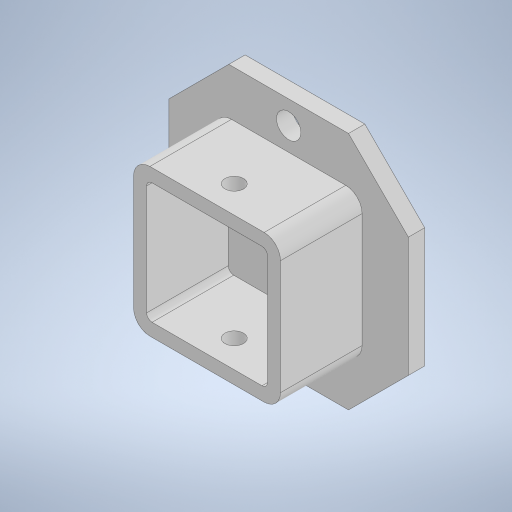
# Autodesk Inventor part: rod_fixture_vp16
Saved by Autodesk Inventor 2024 (Build 280153000, 153)
## iProperties
Created: 2024-10-07
Part Number: rod_fixture_vp16
Material: 一般
Document SubType Name: Modeling
Designer: 1412z
Density: 1 g/cm^3
Appearance: 既定
Author: 1412z
Autodesk Inventor part; units mm, degrees
ref_plane "YZ Plane" through (0, 0, 0) normal (1, 0, 0) x (0, 1, 0)
ref_plane "XZ Plane" through (0, 0, 0) normal (0, 1, 0) x (-1, 0, 0)
ref_plane "XY Plane" through (0, 0, 0) normal (0, 0, 1) x (1, 0, 0)
sketch "スケッチ1" plane through (0, 0, 0) normal (1, 0, 0) x (0, 1, 0)
  point P0 (0, 0)
sketch "スケッチ2" plane through (0, 0, 0) normal (0, 0, 1) x (1, 0, 0)
  line L0 (-11.1, 11.1) -> (11.1, 11.1)
  line L1 (11.1, 11.1) -> (11.1, -11.1)
  line L2 (11.1, -11.1) -> (-11.1, -11.1)
  line L3 (-11.1, -11.1) -> (-11.1, 11.1)
  line L4 (-11.1, 11.1) -> (11.1, -11.1) construction
  line L5 (11.1, 11.1) -> (-11.1, -11.1) construction
  line L6 (-13.5, -13.5) -> (13.5, -13.5)
  line L7 (13.5, -13.5) -> (13.5, 13.5)
  line L8 (13.5, 13.5) -> (-13.5, 13.5)
  line L9 (-13.5, 13.5) -> (-13.5, -13.5)
  line L10 (-13.5, -13.5) -> (13.5, 13.5) construction
  line L11 (13.5, -13.5) -> (-13.5, 13.5) construction
  point P0 (0, 0)
  dimension "d0" = 22.2
  dimension "d1" = 22.2
  dimension "d2" = 27
  dimension "d3" = 27
  constraints: 24 end point, 4 midpoint, 4 parallel, 2 horizontal, 2 perpendicular
  measures "d0" distance of L1.end L2.end
  measures "d1" distance of L0.end L1.end
  measures "d2" distance of L8.end L7.end
  measures "d3" distance of L7.end L6.end
extrude "押し出し1" add sketch "スケッチ2" along normal blind 15
sketch "スケッチ3" plane through (-13.5, 13.5, 0) normal (0, 1, 0) x (1, 0, 0)
  circle A0 centre (13.5, -10) radius 1.7
  point P0 (13.5, 0)
  dimension "d6" = 3.4
  constraints: 1 centre point
  measures "d6" diameter of A0
extrude "押し出し2" cut sketch "スケッチ3" against normal blind 30
sketch "スケッチ4" plane through (0, 0, 0) normal (0, 0, -1) x (-1, 0, 0)
  line L0 (22, 22) -> (-22, 22)
  line L1 (-22, 22) -> (-22, -22)
  line L2 (-22, -22) -> (22, -22)
  line L3 (22, -22) -> (22, 22)
  line L4 (22, 22) -> (-22, -22) construction
  line L5 (-22, 22) -> (22, -22) construction
  point P0 (0, 0)
  dimension "d9" = 44
  dimension "d10" = 44
  constraints: 12 end point, 2 midpoint, 2 parallel, 1 horizontal, 1 perpendicular
  measures "d9" distance of L2.end L1.end
  measures "d10" distance of L1.end L0.end
extrude "押し出し3" add sketch "スケッチ4" along normal blind 3
sketch "スケッチ5" plane through (0, 0, 0) normal (0, 0, 1) x (1, 0, 0)
  circle A0 centre (0, 17.75) radius 2.25
  circle A1 centre (0, -17.75) radius 2.25
  point P0 (0, 0)
  dimension "d13" = 4.5
  dimension "d14" = 4.5
  constraints: 2 centre point
  measures "d13" diameter of A0
  measures "d14" diameter of A1
extrude "押し出し4" cut sketch "スケッチ5" against normal blind 3
sketch "スケッチ6" plane through (0, 0, 0) normal (0, 0, 1) x (1, 0, 0)
  line L0 (-22, 22) -> (22, 22) projected
  line L1 (22, 22) -> (11, 22)
  line L2 (22, 22) -> (22, 11)
  line L3 (22, 11) -> (11, 22)
  line L4 (22, -22) -> (-22, -22) projected
  line L5 (22, -22) -> (22, -11)
  line L6 (22, 22) -> (22, -22) projected
  line L7 (22, -22) -> (11, -22)
  line L8 (11, -22) -> (22, -11)
  line L9 (-22, -22) -> (-22, 22) projected
  line L10 (-22, 22) -> (-11, 22)
  line L11 (-22, 22) -> (-22, 11)
  line L12 (-22, 11) -> (-11, 22)
  line L13 (-22, -22) -> (-22, -11)
  line L14 (-22, -22) -> (-11, -22)
  line L15 (-22, -11) -> (-11, -22)
  point P0 (0, 0)
  dimension "d17" = 11
  dimension "d18" = 11
  dimension "d19" = 11
  dimension "d20" = 11
  dimension "d21" = 11
  dimension "d22" = 11
  dimension "d23" = 11
  constraints: 24 end point, 8 point on line, 1 perpendicular
  measures "d17" distance of L0.end L1.end
  measures "d18" distance of L0.end L2.end
  measures "d19" distance of L4.start L5.end
  measures "d20" distance of L4.start L7.end
  measures "d21" distance of L0.start L10.end
  measures "d22" distance of L0.start L11.end
  measures "d23" distance of L4.end L13.end
extrude "押し出し5" cut sketch "スケッチ6" against normal blind 3 contours L0 L12 L9 | L0 L2 L3 | L15 L4 L9 | L5 L4 L8
fillet "フィレット1" radius 3 4 edges at (13.5, -13.5, 7.5) (13.5, 13.5, 7.5) (-13.5, -13.5, 7.5) (-13.5, 13.5, 7.5)
fillet "フィレット2" radius 1 4 edges at (-11.1, 11.1, 7.5) (-11.1, -11.1, 7.5) (11.1, 11.1, 7.5) (11.1, -11.1, 7.5)
